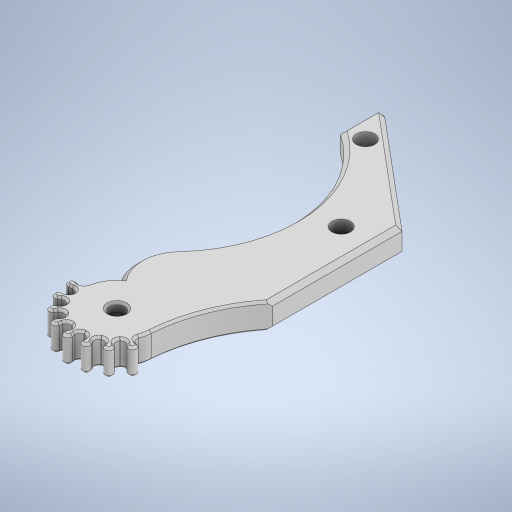
# Autodesk Inventor part: End_Effecto_Claw_R
Saved by Autodesk Inventor 2023 (Build 270158000, 158)
## iProperties
Created: 2025-02-27
Part Number: End_Effecto_Claw_R
Material: Generic
Document SubType Name: Modeling
Designer: Swoby
Density: 1 g/cm^3
Appearance: Default
Author: Swoby
Autodesk Inventor part; units mm, degrees
ref_plane "YZ Plane" through (0, 0, 0) normal (1, 0, 0) x (0, 1, 0)
ref_plane "XZ Plane" through (0, 0, 0) normal (0, 1, 0) x (-1, 0, 0)
ref_plane "XY Plane" through (0, 0, 0) normal (0, 0, 1) x (1, 0, 0)
sketch "Sketch1" plane through (0, 0, 0) normal (0, 1, 0) x (-1, 0, 0)
  line L0 (0, 0) -> (10, 0) construction
  circle A0 centre (10, 0) radius 8.5
  line L1 (0, 0) -> (-10, 0) construction
  circle A1 centre (-10, 0) radius 8.5 construction
  line L2 (10, 0) -> (21.547, -20) construction
  line L3 (21.547, -20) -> (21.547, -40) construction
  line L4 (21.547, -40) -> (0, -65.6787) construction
  line L5 (0, -69.6065) -> (0, -61.751)
  arc A2 (0, -61.751) -> (5.0646, -19.2801) centre (-15.4138, -38.3755) ccw
  line L6 (15.5832, -6.4092) -> (26.547, -19.4754) construction
  line L7 (26.547, -19.4754) -> (26.547, -49.4754)
  line L8 (26.547, -49.4754) -> (1.6428, -70.3725)
  arc A3 (4.4168, -6.4092) -> (5.0646, -19.2801) centre (12.3783, -12.4603) ccw
  arc A4 (5.0646, -19.2801) -> (0, -15) centre (-15.4138, -38.3755) ccw construction
  line L9 (15.5832, -6.4092) -> (4.4168, -6.4092) construction
  arc A5 (18.4809, 0.5693) -> (26.547, -19.4754) centre (53.2139, 2.9008) ccw
  arc A6 (0, -69.6065) -> (1.6428, -70.3725) centre (1, -69.6065) ccw
  circle A7 centre (10, 0) radius 1.75
  circle A8 centre (10, 0) radius 3.4
  point P0 (0, -71.751)
  dimension "d0" = 10
  dimension "d1" = 17
  dimension "d2" = 10
  dimension "d3" = 17
  dimension "d4" = 120
  dimension "d5" = 140
  dimension "d6" = 20
  dimension "d9" = 20
  dimension "d10" = 65.6787
  dimension "d11" = 10
  dimension "d12" = 15
  dimension "d14" = 50
  dimension "d15" = 5
  dimension "d16" = 30
  dimension "d18" = 10
  dimension "d19" = 28
  dimension "d20" = 1
  dimension "d52" = 3.5
  dimension "d53" = 6.8
  constraints: 20 end point, 13 point on circle, 9 centre point, 5 tangent, 4 coincident, 4 point on line, 3 horizontal, 3 vertical, 1 midpoint, 1 perpendicular
  measures "d0" distance of L0.start L0.end
  measures "d1" diameter of A0
  measures "d2" distance of L0.start L1.end
  measures "d3" diameter of A1
  measures "d4" angle of L0 L2
  measures "d5" angle of L3 L4
  measures "d6" distance of L2.end L3.end
  measures "d9" vertical distance of L2.start L2.end
  measures "d10" vertical distance of L4.end L0.end
  measures "d11" distance of point (0, -71.751) L5.end
  measures "d12" distance of L0.start A4.end
  measures "d14" angle of L6 L0
  measures "d15" distance between parallel lines of L3 L7
  measures "d16" distance of L6.end L7.end
  measures "d18" radius of A3
  measures "d19" radius of A2
  measures "d20" radius of A6
  measures "d52" diameter of A7
  measures "d53" diameter of A8
extrude "Extrusion1" add sketch "Sketch1" along normal blind 4 contours A0 | A0 A5 L7 L8 A6 L5 A2 A3 | A8
sketch "Sketch2" plane through (0, 4, 0) normal (0, 1, 0) x (1, 0, 0)
  circle A0 centre (10.329, 0) radius 8.5 construction
  arc A1 (0.2976, -0.877) -> (1.3999, 0) centre (0.4999, 0) ccw
  arc A2 (-1.0376, -3.4403) -> (0.6428, -4.0854) centre (-0.1974, -3.7629) ccw construction
  circle A3 centre (-0.6143, -1.7395) radius 0.9 construction
  line L0 (-10, 0) -> (-18.4288, 0) construction
  line L1 (-10, 0) -> (0.4999, 0) construction
  line L2 (-10, 0) -> (-0.1974, -3.7629) construction
  arc A4 (-0.3792, -0.7208) -> (-1.6423, -1.549) centre (-0.6143, -1.7395) ccw
  line L3 (-0.3792, -0.7208) -> (0.2976, -0.877)
  line L4 (-0.76, -2.7749) -> (-0.072, -2.8716) construction
  arc A5 (-0.4001, 0) -> (0.2976, -0.877) centre (0.4999, 0) ccw construction
  arc A6 (1.3999, 0) -> (0.3757, 0.8914) centre (0.4999, 0) ccw
  arc A7 (-0.072, -2.8716) -> (-1.0376, -3.4403) centre (-0.1974, -3.7629) ccw construction
  arc A8 (0.6428, -4.0854) -> (-0.072, -2.8716) centre (-0.1974, -3.7629) ccw construction
  arc A9 (0.3757, 0.8914) -> (-0.4001, 0) centre (0.4999, 0) ccw construction
  line L5 (-10, 0) -> (-0.6143, -1.7395) construction
  arc A10 (-18.4809, -0.5693) -> (-4.4168, 6.4092) centre (-10, 0) ccw projected
  arc A11 (-1.6423, -1.549) -> (-0.76, -2.7749) centre (-0.6143, -1.7395) ccw construction
  arc A12 (1.3999, 0) -> (0.2976, 0.877) centre (0.4999, 0) ccw
  arc A13 (-1.6423, 1.549) -> (-0.3792, 0.7208) centre (-0.6143, 1.7395) ccw
  line L6 (-0.3792, 0.7208) -> (0.2976, 0.877)
  point P0 (0, 0)
  point P1 (0.3757, 0.8914)
  dimension "d47" = 84
  dimension "d23" = 10
  dimension "d24" = 10.329
  dimension "d26" = 17
  dimension "d36" = 1.8
  dimension "d37" = 1.8
  dimension "d38" = 1.8
  dimension "d39" = 10.4999
  dimension "d40" = 10.5
  dimension "d41" = 21
  dimension "d58" = 10.5
  dimension "d63" = 9.5455
  constraints: 23 point on circle, 14 end point, 13 centre point, 9 tangent, 7 point on line, 4 symmetric about line, 1 coincident, 1 collinear, 1 horizontal, 3 other
  measures "d23" distance of point (-10, 0) point (0, 0)
  measures "d24" distance of A0.centre point (0, 0)
  measures "d26" diameter of A0
  measures "d36" diameter of A1
  measures "d37" diameter of A2
  measures "d38" diameter of A3
  measures "d39" distance of point (-10, 0) L1.end
  measures "d40" distance of point (-10, 0) L2.end
  measures "d41" angle of L2 L1
  measures "d58" angle of L5 L1
  measures "d63" distance of L0.start L5.end
extrude "Extrusion2" add sketch "Sketch2" against normal up to surface (4 mm away)
pattern_circular "Circular Pattern1" count 8 over 149 about axis through (-10, 0, 0) along (0, -1, 0) of "Extrusion2"
mirror "Mirror1" about plane through (0, 0, 0) normal (1, 0, 0) remove original yes
sketch "Sketch3" plane through (26.547, 0, -49.4754) normal (0, -1, 0) x (1, 0, 0)
  arc A0 (-22.1302, 43.0662) -> (-21.4824, 30.1953) centre (-14.1687, 37.0151) ccw projected
  arc A1 (-26.547, -12.2756) -> (-21.4824, 30.1953) centre (-41.9608, 11.0999) ccw projected
  line L0 (-26.547, -12.2756) -> (-26.547, -20.1311) projected
  arc A2 (-26.547, -20.1311) -> (-24.9042, -20.8971) centre (-25.547, -20.1311) ccw projected
  line L1 (-24.9042, -20.8971) -> (0, 0) projected
  line L2 (0, 0) -> (0, 30) projected
  arc A3 (-8.0661, 50.0447) -> (0, 30) centre (26.6669, 52.3762) ccw projected
  arc A4 (-8.0661, 50.0447) -> (-8.5853, 52.4522) centre (-16.547, 49.4754) ccw projected
  arc A5 (-13.1347, 58.4995) -> (-12.6975, 57.0538) centre (-12.224, 57.9859) ccw projected
  line L3 (-12.7935, 59.1045) -> (-13.1347, 58.4995) projected
  arc A6 (-12.7935, 59.1045) -> (-14.4758, 59.6006) centre (-13.5774, 59.5466) ccw projected
  line L4 (-14.5174, 58.9072) -> (-14.4758, 59.6006) projected
  arc A7 (-16.6434, 59.1226) -> (-15.7112, 57.9342) centre (-15.6084, 58.9747) ccw projected
  line L5 (-16.5451, 59.8102) -> (-16.6434, 59.1226) projected
  arc A8 (-16.5451, 59.8102) -> (-18.2927, 59.6617) centre (-17.4361, 59.9376) ccw projected
  line L6 (-18.0798, 59.0006) -> (-18.2927, 59.6617) projected
  arc A9 (-20.139, 58.4295) -> (-18.8389, 57.6606) centre (-19.1209, 58.6674) ccw projected
  line L7 (-20.297, 59.1059) -> (-20.139, 58.4295) projected
  arc A10 (-20.297, 59.1059) -> (-21.8715, 58.3331) centre (-21.1734, 58.9012) ccw projected
  line L8 (-21.4331, 57.7944) -> (-21.8715, 58.3331) projected
  arc A11 (-23.1445, 56.5147) -> (-21.654, 56.2702) centre (-22.2821, 57.1059) ccw projected
  line L9 (-23.5372, 57.0876) -> (-23.1445, 56.5147) projected
  arc A12 (-23.5372, 57.0876) -> (-24.7237, 55.796) centre (-24.2795, 56.5787) ccw projected
  line L10 (-24.1197, 55.4531) -> (-24.7237, 55.796) projected
  arc A13 (-25.2498, 53.6395) -> (-23.7722, 53.9527) centre (-24.6609, 54.5034) ccw projected
  line L11 (-25.8237, 54.0307) -> (-25.2498, 53.6395) projected
  arc A14 (-25.8237, 54.0307) -> (-26.4604, 52.3965) centre (-26.3306, 53.2871) ccw projected
  line L12 (-25.7731, 52.2963) -> (-26.4604, 52.3965) projected
  arc A15 (-26.1678, 50.1962) -> (-24.9047, 51.0244) centre (-25.9327, 51.2149) ccw projected
  line L13 (-26.8446, 50.3523) -> (-26.1678, 50.1962) projected
  arc A16 (-26.8446, 50.3523) -> (-26.8446, 48.5984) centre (-27.0469, 49.4754) ccw projected
  line L14 (-26.1678, 48.7546) -> (-26.8446, 48.5984) projected
  arc A17 (-24.9047, 47.9264) -> (-26.1678, 48.7546) centre (-25.9327, 47.7359) ccw projected
  arc A18 (-24.9047, 47.9264) -> (-22.1302, 43.0662) centre (-16.547, 49.4754) ccw projected
  circle A19 centre (-16.547, 49.4754) radius 1.75 projected
  arc A20 (-13.0333, 50.7855) -> (-19.8092, 47.6258) centre (-16.547, 49.4754) ccw
  line L15 (-16.547, 49.4754) -> (-9.8908, 35.201) construction
  arc A21 (-12.0655, 33.968) -> (-7.5483, 36.0744) centre (-9.8908, 35.201) ccw
  line L16 (-13.0333, 50.7855) -> (-7.5483, 36.0744)
  line L17 (-19.8092, 47.6258) -> (-12.0655, 33.968)
  line L18 (-16.5263, 49.431) -> (-18.1318, 52.874) construction
  line L19 (-9.8908, 35.201) -> (-8.8342, 32.9353) construction
  arc A22 (-14.9622, 46.0767) -> (-13.0333, 50.7855) centre (-16.547, 49.4754) ccw construction
  arc A23 (-19.8092, 47.6258) -> (-14.9622, 46.0767) centre (-16.547, 49.4754) ccw construction
  arc A24 (-10.9473, 37.4668) -> (-12.0655, 33.968) centre (-9.8908, 35.201) ccw construction
  arc A25 (-7.5483, 36.0744) -> (-10.9473, 37.4668) centre (-9.8908, 35.201) ccw construction
  arc A26 (-7.9292, 53.8126) -> (-8.5853, 52.4522) centre (-7.606, 52.8183) ccw projected
  line L20 (-7.2686, 54.0273) -> (-7.9292, 53.8126) projected
  arc A27 (-7.2686, 54.0273) -> (-8.1719, 55.5307) centre (-7.5468, 54.8833) ccw projected
  line L21 (-8.6716, 55.0483) -> (-8.1719, 55.5307) projected
  arc A28 (-10.1809, 55.1077) -> (-8.6716, 55.0483) centre (-9.3978, 55.8004) ccw projected
  arc A29 (-10.1809, 55.1077) -> (-10.209, 55.1393) centre (-16.547, 49.4754) ccw projected
  arc A30 (-10.0916, 56.6452) -> (-10.209, 55.1393) centre (-9.4295, 55.836) ccw projected
  line L22 (-9.554, 57.085) -> (-10.0916, 56.6452) projected
  arc A31 (-9.554, 57.085) -> (-10.9415, 58.1579) centre (-10.1239, 57.7816) ccw projected
  line L23 (-11.2319, 57.527) -> (-10.9415, 58.1579) projected
  arc A32 (-12.6598, 57.0345) -> (-11.2319, 57.527) centre (-12.1816, 57.9643) ccw projected
  arc A33 (-12.6598, 57.0345) -> (-12.6975, 57.0538) centre (-16.547, 49.4754) ccw projected
  arc A34 (-15.6691, 57.9299) -> (-14.5174, 58.9072) centre (-15.5611, 58.9699) ccw projected
  arc A35 (-15.6691, 57.9299) -> (-15.7112, 57.9342) centre (-16.547, 49.4754) ccw projected
  arc A36 (-18.7981, 57.6719) -> (-18.0798, 59.0006) centre (-19.075, 58.6801) ccw projected
  arc A37 (-18.7981, 57.6719) -> (-18.8389, 57.6606) centre (-16.547, 49.4754) ccw projected
  arc A38 (-21.62, 56.2955) -> (-21.4331, 57.7944) centre (-22.244, 57.1344) ccw projected
  arc A39 (-21.62, 56.2955) -> (-21.654, 56.2702) centre (-16.547, 49.4754) ccw projected
  arc A40 (-23.7498, 53.9887) -> (-24.1197, 55.4531) centre (-24.6358, 54.5438) ccw projected
  arc A41 (-23.7498, 53.9887) -> (-23.7722, 53.9527) centre (-16.547, 49.4754) ccw projected
  arc A42 (-24.8968, 51.0661) -> (-25.7731, 52.2963) centre (-25.9239, 51.2617) ccw projected
  arc A43 (-24.8968, 51.0661) -> (-24.9047, 51.0244) centre (-16.547, 49.4754) ccw projected
  point P0 (-26.547, 49.4754)
  dimension "d67" = 7.5
  dimension "d68" = 25
  dimension "d69" = 22
  dimension "d70" = 5
  constraints: 16 point on circle, 10 end point, 8 tangent, 6 centre point, 3 point on line, 2 coincident, 2 collinear
  measures "d67" diameter of A20
  measures "d68" angle of L2 L15
  measures "d69" distance of L19.end L18.end
  measures "d70" diameter of A21
sketch "Sketch4" plane through (-0.4999, 4, 0) normal (0, 1, 0) x (1, 0, 0)
  arc A0 (5.5645, 19.2801) -> (4.9167, 6.4092) centre (12.8782, 12.4603) ccw projected
  arc A1 (4.9167, 6.4092) -> (2.1423, 1.549) centre (10.4999, 0) ccw projected
  arc A2 (0.8792, 0.7208) -> (2.1423, 1.549) centre (1.1142, 1.7395) ccw projected
  line L0 (0.2024, 0.877) -> (0.8792, 0.7208) projected
  arc A3 (0.2024, 0.877) -> (0.2024, -0.877) centre (0, 0) ccw projected
  line L1 (0.8792, -0.7208) -> (0.2024, -0.877) projected
  arc A4 (2.1423, -1.549) -> (0.8792, -0.7208) centre (1.1142, -1.7395) ccw projected
  line L2 (0.5865, -2.9211) -> (1.2738, -2.8209) projected
  arc A5 (0.5865, -2.9211) -> (1.2232, -4.5553) centre (0.7163, -3.8117) ccw projected
  line L3 (1.7971, -4.1641) -> (1.2232, -4.5553) projected
  arc A6 (3.2747, -4.4773) -> (1.7971, -4.1641) centre (2.386, -5.028) ccw projected
  line L4 (2.3232, -6.3206) -> (2.9272, -5.9777) projected
  arc A7 (2.3232, -6.3206) -> (3.5097, -7.6122) centre (2.7674, -7.1033) ccw projected
  line L5 (3.9025, -7.0393) -> (3.5097, -7.6122) projected
  arc A8 (5.393, -6.7948) -> (3.9025, -7.0393) centre (4.7648, -7.6306) ccw projected
  line L6 (5.1755, -8.8577) -> (5.6139, -8.319) projected
  arc A9 (5.1755, -8.8577) -> (6.7499, -9.6305) centre (5.8735, -9.4258) ccw projected
  line L7 (6.9079, -8.9541) -> (6.7499, -9.6305) projected
  arc A10 (8.208, -8.1852) -> (6.9079, -8.9541) centre (7.9261, -9.192) ccw projected
  line L8 (8.7542, -10.1863) -> (8.9671, -9.5252) projected
  arc A11 (8.7542, -10.1863) -> (10.5018, -10.3348) centre (9.6109, -10.4622) ccw projected
  line L9 (10.4035, -9.6473) -> (10.5018, -10.3348) projected
  arc A12 (11.3357, -8.4588) -> (10.4035, -9.6473) centre (11.4385, -9.4993) ccw projected
  line L10 (12.5711, -10.1252) -> (12.5295, -9.4318) projected
  arc A13 (12.5711, -10.1252) -> (14.2534, -9.6291) centre (13.4695, -10.0712) ccw projected
  line L11 (13.9122, -9.0241) -> (14.2534, -9.6291) projected
  arc A14 (14.3494, -7.5784) -> (13.9122, -9.0241) centre (14.8229, -8.5105) ccw projected
  arc A15 (18.4616, -2.9768) -> (18.9808, -0.5693) centre (10.4999, 0) ccw projected
  arc A16 (27.0469, 19.4754) -> (18.9808, -0.5693) centre (53.7138, -2.9008) ccw projected
  line L12 (27.0469, 49.4754) -> (27.0469, 19.4754) projected
  line L13 (2.1427, 70.3725) -> (27.0469, 49.4754) projected
  arc A17 (2.1427, 70.3725) -> (0.4999, 69.6065) centre (1.4999, 69.6065) ccw projected
  line L14 (0.4999, 61.751) -> (0.4999, 69.6065) projected
  arc A18 (5.5645, 19.2801) -> (0.4999, 61.751) centre (-14.9139, 38.3755) ccw projected
  circle A19 centre (10.4999, 0) radius 1.75 projected
  line L15 (4.9167, 6.4092) -> (16.6597, 26.7486)
  arc A20 (27.0469, 19.4754) -> (27.0469, 27.6574) centre (22.1715, 23.5664) ccw construction
  arc A21 (27.0469, 27.6574) -> (16.6597, 26.7486) centre (22.1715, 23.5664) ccw
  arc A22 (2.1423, -1.549) -> (2.1501, -1.5907) centre (10.4999, 0) ccw projected
  arc A23 (1.2738, -2.8209) -> (2.1501, -1.5907) centre (1.123, -1.7863) ccw projected
  arc A24 (3.2747, -4.4773) -> (3.2971, -4.5133) centre (10.4999, 0) ccw projected
  arc A25 (2.9272, -5.9777) -> (3.2971, -4.5133) centre (2.4112, -5.0684) ccw projected
  arc A26 (5.393, -6.7948) -> (5.4269, -6.8202) centre (10.4999, 0) ccw projected
  arc A27 (5.6139, -8.319) -> (5.4269, -6.8202) centre (4.8029, -7.6591) ccw projected
  arc A28 (8.208, -8.1852) -> (8.2488, -8.1965) centre (10.4999, 0) ccw projected
  arc A29 (8.9671, -9.5252) -> (8.2488, -8.1965) centre (7.9719, -9.2047) ccw projected
  arc A30 (11.3357, -8.4588) -> (11.3779, -8.4545) centre (10.4999, 0) ccw projected
  arc A31 (12.5295, -9.4318) -> (11.3779, -8.4545) centre (11.4859, -9.4945) ccw projected
  arc A32 (14.3494, -7.5784) -> (14.3871, -7.5591) centre (10.4999, 0) ccw projected
  arc A33 (15.815, -8.0516) -> (14.3871, -7.5591) centre (14.8653, -8.4889) ccw projected
  line L16 (16.1055, -8.6826) -> (15.815, -8.0516) projected
  arc A34 (16.1055, -8.6826) -> (17.4929, -7.6096) centre (16.923, -8.3062) ccw projected
  line L17 (16.9554, -7.1698) -> (17.4929, -7.6096) projected
  arc A35 (16.8379, -5.6639) -> (16.9554, -7.1698) centre (17.6175, -6.3606) ccw projected
  arc A36 (16.8379, -5.6639) -> (16.866, -5.6323) centre (10.4999, 0) ccw projected
  arc A37 (18.3753, -5.5729) -> (16.866, -5.6323) centre (17.6491, -6.3251) ccw projected
  line L18 (18.875, -6.0553) -> (18.3753, -5.5729) projected
  arc A38 (18.875, -6.0553) -> (19.7783, -4.5519) centre (19.5001, -5.4079) ccw projected
  line L19 (19.1178, -4.3372) -> (19.7783, -4.5519) projected
  arc A39 (18.4616, -2.9768) -> (19.1178, -4.3372) centre (19.441, -3.3429) ccw projected
  point P0 (0.4999, 0)
  dimension "d72" = 150
  constraints: 4 point on circle, 3 tangent, 2 centre point, 2 end point, 1 point on line
  measures "d72" angle of L15 L12
extrude "Extrusion5" add sketch "Sketch4" along normal blind 2
extrude "Extrusion6" cut sketch "Sketch3" against normal blind 4 contours L16 A21 L17 A20
chamfer "Chamfer1" distance 1 angle 45 12 edges at (12.3892, 0, -41.6909) (2.3909, 0, -12.9629) (14.0949, 0, -59.924) (0.5774, 0, -70.5128) (0, 0, -65.6787) (26.547, 0, -34.4754) (26.547, 6, -34.4754) (12.3892, 6, -41.6909) (2.3909, 6, -12.9629) (14.0949, 6, -59.924) (0.5774, 6, -70.5128) (0, 6, -65.6787)
chamfer "Chamfer2" distance 0.5 angle 45 111 edges at (8.25, 6, 0) (20.6293, 6, -9.3492) (18.309, 6, 1.7919) (17.9993, 6, 3.7971) (18.9481, 6, 4.4446) (19.7716, 6, 5.8714) (18.1252, 6, 5.8141) (17.1081, 6, 5.2803) (16.3521, 6, 5.6481) (16.0752, 6, 6.442) (16.7242, 6, 7.3897) (16.9736, 6, 9.0181) (15.4603, 6, 8.3671) (14.7063, 6, 7.5005) (13.8684, 6, 7.5687) (13.3222, 6, 8.2079) (13.5829, 6, 9.3266) (13.2241, 6, 10.9345) (12.0504, 6, 9.7785) (11.6624, 6, 8.6973) (10.8569, 6, 8.4567) (10.1159, 6, 8.854) (9.9527, 6, 9.991) (9.0347, 6, 11.359) (8.3607, 6, 9.8558) (8.3917, 6, 8.7075) (7.7285, 6, 8.1909) (6.8939, 6, 8.2921) (6.329, 6, 9.2923) (4.9771, 6, 10.2337) (4.8947, 6, 8.5883) (5.3405, 6, 7.5296) (4.91, 6, 6.8075) (4.0956, 6, 6.5988) (3.2062, 6, 7.3258) (1.6047, 6, 7.7121) (2.1253, 6, 6.1491) (2.9249, 6, 5.3245) (2.786, 6, 4.4953) (2.1029, 6, 4.0052) (1.0102, 6, 4.3597) (-0.6222, 6, 4.1384) (0.4302, 6, 2.871) (1.4747, 6, 2.3929) (1.6462, 6, 1.5698) (1.1876, 6, 0.8652) (0.0408, 6, 0.7989) (-1.3999, 6, 0) (0.0408, 6, -0.7989) (1.1876, 6, -0.8652) (4.8035, 6, -6.7265) (2.6181, 6, -4.214) (20.6293, 0, -9.3492) (18.309, 0, 1.7919) (17.9993, 0, 3.7971) (18.9481, 0, 4.4446) (19.7913, 0, 5.8369) (18.4042, 0, 6.0823) (18.1252, 0, 5.8141) (17.1081, 0, 5.2803) (16.3521, 0, 5.6481) (16.0752, 0, 6.442) (16.7242, 0, 7.3897) (17.0045, 0, 8.9932) (15.6229, 0, 8.7183) (15.4603, 0, 8.3671) (14.7063, 0, 7.5005) (13.8684, 0, 7.5687) (13.3222, 0, 8.2079) (13.5829, 0, 9.3266) (13.262, 0, 10.9224) (12.0745, 0, 10.1647) (12.0504, 0, 9.7785) (11.6624, 0, 8.6973) (10.8569, 0, 8.4567) (10.1159, 0, 8.854) (9.9527, 0, 9.991) (9.0744, 0, 11.3615) (8.2429, 0, 10.2244) (8.3607, 0, 9.8558) (8.3917, 0, 8.7075) (7.7285, 0, 8.1909) (6.8939, 0, 8.2921) (6.329, 0, 9.2923) (4.6512, 0, 8.8891) (5.0131, 0, 10.2504) (4.8947, 0, 8.5883) (5.3405, 0, 7.5296) (4.91, 0, 6.8075) (4.0956, 0, 6.5988) (3.2062, 0, 7.3258) (1.7892, 0, 6.3409) (1.6322, 0, 7.7408) (2.1253, 0, 6.1491) (2.9249, 0, 5.3245) (2.786, 0, 4.4953) (2.1029, 0, 4.0052) (1.0102, 0, 4.3597) (0.0474, 0, 2.9277) (-0.607, 0, 4.1751) (0.4302, 0, 2.871) (1.4747, 0, 2.3929) (1.6462, 0, 1.5698) (1.1876, 0, 0.8652) (0.0408, 0, 0.7989) (-0.3364, 0, -0.885) (-1.399, 0, 0.0397) (0.0408, 0, -0.7989) (1.1876, 0, -0.8652) (4.8035, 0, -6.7265) (2.6181, 0, -4.214)
sketch "Sketch5" plane through (-0.4999, 6, 0) normal (0, 1, 0) x (1, 0, 0)
  arc A0 (26.0469, 19.0405) -> (18.482, -0.5358) centre (53.7138, -2.9008) ccw projected
  line L0 (26.0469, 49.0091) -> (26.0469, 19.0405) projected
  line L1 (1.4999, 69.6065) -> (26.0469, 49.0091) projected
  line L2 (1.4999, 62.2833) -> (1.4999, 69.6065) projected
  arc A1 (6.2958, 18.5981) -> (1.4999, 62.2833) centre (-14.9139, 38.3755) ccw projected
  arc A2 (6.2958, 18.5981) -> (6.0223, 6.6296) centre (12.8782, 12.4603) ccw projected
  arc A3 (6.0223, 6.6296) -> (2.6339, 1.4579) centre (10.4999, 0) ccw projected
  arc A4 (0.7667, 0.2336) -> (2.6339, 1.4579) centre (1.1142, 1.7395) ccw projected
  line L3 (0.0899, 0.3898) -> (0.7667, 0.2336) projected
  arc A5 (0.0899, 0.3898) -> (0.0899, -0.3898) centre (0, 0) ccw projected
  line L4 (0.7667, -0.2336) -> (0.0899, -0.3898) projected
  arc A6 (2.6339, -1.4579) -> (0.7667, -0.2336) centre (1.1142, -1.7395) ccw projected
  arc A7 (2.6339, -1.4579) -> (2.6413, -1.4971) centre (10.4999, 0) ccw projected
  arc A8 (1.3459, -3.3157) -> (2.6413, -1.4971) centre (1.123, -1.7863) ccw projected
  line L5 (0.6586, -3.4159) -> (1.3459, -3.3157) projected
  arc A9 (0.6586, -3.4159) -> (0.9416, -4.1422) centre (0.7163, -3.8117) ccw projected
  line L6 (1.5155, -3.751) -> (0.9416, -4.1422) projected
  arc A10 (3.6997, -4.214) -> (1.5155, -3.751) centre (2.386, -5.028) ccw projected
  arc A11 (3.6997, -4.214) -> (3.7208, -4.2478) centre (10.4999, 0) ccw projected
  arc A12 (3.174, -6.4126) -> (3.7208, -4.2478) centre (2.4112, -5.0684) ccw projected
  line L7 (2.57, -6.7554) -> (3.174, -6.4126) projected
  arc A13 (2.57, -6.7554) -> (3.0973, -7.3295) centre (2.7674, -7.1033) ccw projected
  line L8 (3.4901, -6.7566) -> (3.0973, -7.3295) projected
  arc A14 (5.6934, -6.3951) -> (3.4901, -6.7566) centre (4.7648, -7.6306) ccw projected
  arc A15 (5.6934, -6.3951) -> (5.7253, -6.419) centre (10.4999, 0) ccw projected
  arc A16 (6.0017, -8.6346) -> (5.7253, -6.419) centre (4.8029, -7.6591) ccw projected
  line L9 (5.5633, -9.1733) -> (6.0017, -8.6346) projected
  arc A17 (5.5633, -9.1733) -> (6.2631, -9.5168) centre (5.8735, -9.4258) ccw projected
  line L10 (6.4211, -8.8404) -> (6.2631, -9.5168) projected
  arc A18 (8.3428, -7.7037) -> (6.4211, -8.8404) centre (7.9261, -9.192) ccw projected
  arc A19 (8.3428, -7.7037) -> (8.3812, -7.7144) centre (10.4999, 0) ccw projected
  arc A20 (9.4431, -9.6785) -> (8.3812, -7.7144) centre (7.9719, -9.2047) ccw projected
  line L11 (9.2301, -10.3396) -> (9.4431, -9.6785) projected
  arc A21 (9.2301, -10.3396) -> (10.0068, -10.4056) centre (9.6109, -10.4622) ccw projected
  line L12 (9.9085, -9.718) -> (10.0068, -10.4056) projected
  arc A22 (11.2865, -7.9612) -> (9.9085, -9.718) centre (11.4385, -9.4993) ccw projected
  arc A23 (11.2865, -7.9612) -> (11.3262, -7.9572) centre (10.4999, 0) ccw projected
  arc A24 (13.0286, -9.4019) -> (11.3262, -7.9572) centre (11.4859, -9.4945) ccw projected
  line L13 (13.0702, -10.0952) -> (13.0286, -9.4019) projected
  arc A25 (13.0702, -10.0952) -> (13.8179, -9.8747) centre (13.4695, -10.0712) ccw projected
  line L14 (13.4767, -9.2698) -> (13.8179, -9.8747) projected
  arc A26 (14.123, -7.1326) -> (13.4767, -9.2698) centre (14.8229, -8.5105) ccw projected
  arc A27 (14.123, -7.1326) -> (14.1585, -7.1144) centre (10.4999, 0) ccw projected
  arc A28 (16.2692, -7.8425) -> (14.1585, -7.1144) centre (14.8653, -8.4889) ccw projected
  line L15 (16.5596, -8.4735) -> (16.2692, -7.8425) projected
  arc A29 (16.5596, -8.4735) -> (17.1763, -7.9966) centre (16.923, -8.3062) ccw projected
  line L16 (16.6387, -7.5568) -> (17.1763, -7.9966) projected
  arc A30 (16.4651, -5.3308) -> (16.6387, -7.5568) centre (17.6175, -6.3606) ccw projected
  arc A31 (16.4651, -5.3308) -> (16.4916, -5.301) centre (10.4999, 0) ccw projected
  arc A32 (18.7226, -5.2132) -> (16.4916, -5.301) centre (17.6491, -6.3251) ccw projected
  line L17 (19.2223, -5.6956) -> (18.7226, -5.2132) projected
  arc A33 (19.2223, -5.6956) -> (19.6238, -5.0274) centre (19.5001, -5.4079) ccw projected
  line L18 (18.9632, -4.8127) -> (19.6238, -5.0274) projected
  arc A34 (17.9933, -2.8017) -> (18.9632, -4.8127) centre (19.441, -3.3429) ccw projected
  arc A35 (17.9933, -2.8017) -> (18.482, -0.5358) centre (10.4999, 0) ccw projected
  circle A36 centre (10.4999, 0) radius 2.25 projected
  arc A37 (5.5645, 19.2801) -> (0.4999, 61.751) centre (-14.9139, 38.3755) ccw projected
  line L19 (5.5645, 19.2801) -> (6.2958, 18.5981) projected
  arc A38 (6.2958, 18.5981) -> (1.4999, 62.2833) centre (-14.9139, 38.3755) ccw projected
  line L20 (1.4999, 62.2833) -> (1.4999, 69.6065) projected
  line L21 (1.4999, 69.6065) -> (0.4999, 69.6065) projected
  line L22 (0.4999, 69.6065) -> (0.4999, 61.751) projected
  arc A39 (27.0469, 19.4754) -> (26.5469, 18.8656) centre (53.7138, -2.9008) ccw projected
  line L23 (27.0469, 19.4754) -> (27.0469, 49.4754) projected
  line L24 (26.0469, 49.0091) -> (27.0469, 49.4754) projected
  line L25 (26.0469, 49.0091) -> (26.0469, 19.0405) projected
  line L26 (27.0469, 49.4754) -> (2.1427, 70.3725) projected
  line L27 (2.1427, 70.3725) -> (1.4999, 69.6065) projected
  line L28 (1.4999, 69.6065) -> (26.0469, 49.0091) projected
  line L29 (26.0469, 49.0091) -> (27.0469, 49.4754) projected
  line L30 (1.4999, 69.6065) -> (0.4999, 69.6065) projected
  line L31 (2.1427, 70.3725) -> (1.4999, 69.6065) projected
  arc A40 (2.1427, 70.3725) -> (0.4999, 69.6065) centre (1.4999, 69.6065) ccw projected
  line L32 (1.4999, 65.9449) -> (20.0665, 50.3657) construction
  line L33 (20.0665, 50.3657) -> (20.0665, 22.4985) construction
  circle A41 centre (5.3301, 62.731) radius 2.15
  circle A42 centre (20.0665, 42.3657) radius 2.15
  point P0 (0.4999, 0)
  dimension "d83" = 11.9609
  dimension "d84" = 5.9804
  dimension "d85" = 4.3
  dimension "d86" = 4.3
  dimension "d87" = 8
  dimension "d88" = 5
  constraints: 4 end point, 2 centre point, 2 midpoint, 2 parallel, 2 point on line, 3 other
  measures "d83" distance edge to line of A1 L0
  measures "d84" distance between parallel lines of L33 L0
  measures "d85" diameter of A41
  measures "d86" diameter of A42
  measures "d87" distance of L32.end A42.centre
  measures "d88" distance of A41.centre point (1.5, 65.945)
extrude "Extrusion7" cut sketch "Sketch5" against normal through all contours A41 | A42
equation "\"d3\" = d1"
equation "\"d26\" = 2 * d25"
equation "\"d58\" = 0.5 * d41"
equation "\"d84\" = 0.5 * d83"
equation "\"d25\" = 8.5"
body "Solid1"
